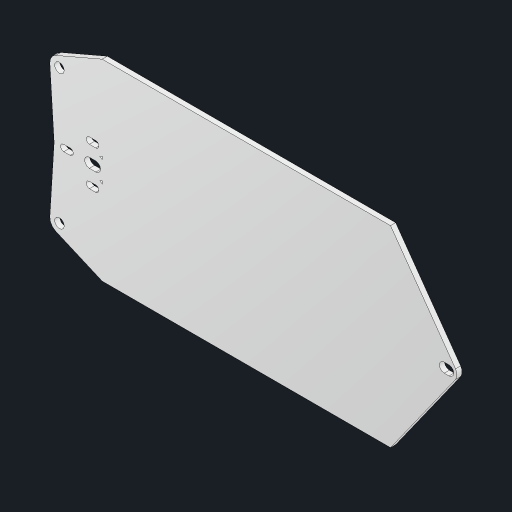
# Autodesk Inventor part: Bottom Plate Poly
Saved by Autodesk Inventor 2023.2 (Build 272271030, 271C)
## iProperties
Created: 2024-02-28
Part Number: Bottom Plate Poly
Material: Aluminum 6061
Document SubType Name: Modeling
Designer: robpl
Density: 2.7 g/cm^3
Appearance: Aluminum - Flat
Mass: 11.953 g
Surface Area: 75.4446 cm^2
Volume: 4.42704 cm^3
Author: robpl
Autodesk Inventor part; units mm, degrees
ref_plane "YZ Plane" through (0, 0, 0) normal (1, 0, 0) x (0, 1, 0)
ref_plane "XZ Plane" through (0, 0, 0) normal (0, 1, 0) x (-1, 0, 0)
ref_plane "XY Plane" through (0, 0, 0) normal (0, 0, 1) x (1, 0, 0)
sketch "Sketch1" plane through (0, 0, 0) normal (0, 0, 1) x (1, 0, 0)
  line L0 (-45, 25) -> (45, 25)
  line L1 (45, 25) -> (45, -25)
  line L2 (45, -25) -> (-45, -25)
  line L3 (-45, -25) -> (-45, 25)
  line L4 (-45, 25) -> (45, -25) construction
  line L5 (45, 25) -> (-45, -25) construction
  line L6 (-45, -25) -> (-40, -25)
  line L7 (-40, -25) -> (-40, -47)
  line L8 (-40, -47) -> (-45, -47)
  line L9 (-45, -47) -> (-45, -25)
  line L10 (45, -25) -> (40, -25)
  line L11 (40, -25) -> (40, -47)
  line L12 (40, -47) -> (45, -47)
  line L13 (45, -47) -> (45, -25)
  line L14 (45, 25) -> (40, 25)
  line L15 (40, 25) -> (40, 47)
  line L16 (40, 47) -> (45, 47)
  line L17 (45, 47) -> (45, 25)
  line L18 (-45, 25) -> (-40, 25)
  line L19 (-40, 25) -> (-40, 47)
  line L20 (-40, 47) -> (-45, 47)
  line L21 (-45, 47) -> (-45, 25)
  circle A0 centre (-48, 0) radius 18
  circle A1 centre (0, 0) radius 66
  circle A2 centre (-58.3352, 21) radius 4
  circle A3 centre (-58.3352, -21) radius 4
  circle A4 centre (-58.3352, -21) radius 1.5
  circle A5 centre (-58.3352, 21) radius 1.5
  line L22 (61.75, 0) -> (63.25, 0) construction
  line L23 (61.75, -4) -> (63.25, -4)
  line L24 (63.25, 4) -> (61.75, 4)
  arc A6 (61.75, 4) -> (61.75, -4) centre (61.75, 0) ccw
  arc A7 (63.25, -4) -> (63.25, 4) centre (63.25, 0) ccw
  line L25 (61.75, 0) -> (63.25, 0) construction
  line L26 (61.75, -1.5) -> (63.25, -1.5)
  line L27 (63.25, 1.5) -> (61.75, 1.5)
  arc A8 (61.75, 1.5) -> (61.75, -1.5) centre (61.75, 0) ccw
  arc A9 (63.25, -1.5) -> (63.25, 1.5) centre (63.25, 0) ccw
  circle A10 centre (61.75, 0) radius 4.25 construction
  circle A11 centre (61.75, 0) radius 4 construction
  line L28 (-45, -25) -> (45, -25) construction
  line L29 (45, -25) -> (45, -30) construction
  line L30 (45, -30) -> (-45, -30)
  line L31 (-45, -30) -> (-45, -25) construction
  line L32 (-45, 30) -> (45, 30)
  line L33 (-47, 0) -> (-49, 0) construction
  line L34 (-47, 1.5) -> (-49, 1.5)
  line L35 (-49, -1.5) -> (-47, -1.5)
  arc A12 (-47, -1.5) -> (-47, 1.5) centre (-47, 0) ccw
  arc A13 (-49, 1.5) -> (-49, -1.5) centre (-49, 0) ccw
  line L36 (-40, 0) -> (-56, 0) construction
  line L37 (-48, -6) -> (-48, 6) construction
  line L38 (-47, 6) -> (-49, 6) construction
  line L39 (-47, 7) -> (-49, 7)
  line L40 (-49, 5) -> (-47, 5)
  arc A14 (-47, 5) -> (-47, 7) centre (-47, 6) ccw
  arc A15 (-49, 7) -> (-49, 5) centre (-49, 6) ccw
  line L41 (-55, 0) -> (-57, 0) construction
  line L42 (-55, 1) -> (-57, 1)
  line L43 (-57, -1) -> (-55, -1)
  arc A16 (-55, -1) -> (-55, 1) centre (-55, 0) ccw
  arc A17 (-57, 1) -> (-57, -1) centre (-57, 0) ccw
  line L44 (-47, -6) -> (-49, -6) construction
  line L45 (-47, -5) -> (-49, -5)
  line L46 (-49, -7) -> (-47, -7)
  arc A18 (-47, -7) -> (-47, -5) centre (-47, -6) ccw
  arc A19 (-49, -5) -> (-49, -7) centre (-49, -6) ccw
  line L47 (-49, 3) -> (-47, 3)
  arc A20 (-47, 3) -> (-47, 9) centre (-47, 6) ccw
  line L48 (-47, 9) -> (-49, 9)
  arc A21 (-49, 9) -> (-49, 3) centre (-49, 6) ccw
  line L49 (-49, -3.5) -> (-47, -3.5)
  arc A22 (-47, -3.5) -> (-47, 3.5) centre (-47, 0) ccw
  line L50 (-47, 3.5) -> (-49, 3.5)
  arc A23 (-49, 3.5) -> (-49, -3.5) centre (-49, 0) ccw
  line L51 (-49, -9) -> (-47, -9)
  arc A24 (-47, -9) -> (-47, -3) centre (-47, -6) ccw
  line L52 (-47, -3) -> (-49, -3)
  arc A25 (-49, -3) -> (-49, -9) centre (-49, -6) ccw
  line L53 (-57, -3) -> (-55, -3)
  arc A26 (-55, -3) -> (-55, 3) centre (-55, 0) ccw
  line L54 (-55, 3) -> (-57, 3)
  arc A27 (-57, 3) -> (-57, -3) centre (-57, 0) ccw
  line L55 (-40, 25) -> (-44.0624, 5.3914)
  line L56 (-40, -25) -> (-44.0624, -5.3914)
  line L57 (61.75, -2.5) -> (63.25, -2.5)
  arc A28 (63.25, -2.5) -> (63.25, 2.5) centre (63.25, 0) ccw
  line L58 (63.25, 2.5) -> (61.75, 2.5)
  arc A29 (61.75, 2.5) -> (61.75, -2.5) centre (61.75, 0) ccw
  line L59 (65.2879, -1.4481) -> (45, -30)
  line L60 (45, 30) -> (65.2879, 1.4481)
  line L61 (42.4191, 25) -> (59.464, 1.0121)
  line L62 (42.4191, -25) -> (59.464, -1.0121)
  circle A30 centre (-58.3352, -21) radius 3
  circle A31 centre (-58.3352, 21) radius 3
  line L63 (-45, -30) -> (-59.5204, -23.756)
  line L64 (-45, 30) -> (-59.5204, 23.756)
  line L65 (-60, 0) -> (-61.3291, -20.8088)
  line L66 (-60, 0) -> (-61.3291, 20.8088)
  point P0 (62.5, 0)
  point P1 (62.5, 0)
  point P2 (-45.7543, -3.2708)
  point P3 (-45.7543, 3.2708)
  point P4 (58.5132, -2.3502)
  point P5 (58.5132, 2.3502)
  point P6 (-45, 3.7639)
  point P7 (-45, 2.8723)
  point P8 (-45, -2.8723)
  point P9 (-45, -3.7639)
  dimension "d0" = 90
  dimension "d1" = 50
  dimension "d2" = 5
  dimension "d3" = 22
  dimension "d5" = 36
  dimension "d6" = 132
  dimension "d7" = 8
  dimension "d8" = 8
  dimension "d9" = 4
  dimension "d10" = 3
  dimension "d11" = 3
  dimension "d12" = 8
  dimension "d13" = 3
  dimension "d14" = 1.5
  dimension "d15" = 8.5
  dimension "d16" = 1.25
  dimension "d17" = 5
  dimension "d18" = 5
  dimension "d19" = 1
  dimension "d20" = 3
  dimension "d21" = 16
  dimension "d22" = 12
  dimension "d23" = 1
  dimension "d24" = 1
  dimension "d25" = 1
  dimension "d26" = 2
  dimension "d27" = 1
  dimension "d28" = 2
  dimension "d29" = 2
  dimension "d30" = 2
  dimension "d31" = 2
  dimension "d32" = 2
  dimension "d33" = 1
  dimension "d35" = 5
  dimension "d36" = 5
  dimension "d37" = 1.5
  dimension "d38" = 1.5
  constraints: 146 end point, 55 point on circle, 36 tangent, 31 centre point, 26 parallel, 11 horizontal, 10 midpoint, 8 perpendicular, 6 coincident, 6 point on line, 5 equal length, 2 horizontal alignment, 2 vertical alignment, 1 collinear, 17 other
  measures "d0" distance of L1.end L2.end
  measures "d1" distance of L0.end L1.end
  measures "d2" distance of L7.end L8.end
  measures "d3" distance of L6.end L7.end
  measures "d5" diameter of A0
  measures "d6" diameter of A1
  measures "d7" diameter of A2
  measures "d8" diameter of A3
  measures "d9" distance from line of A2.centre L0
  measures "d10" diameter of A4
  measures "d11" diameter of A5
  measures "d12" diameter of A7
  measures "d13" diameter of A9
  measures "d14" distance of L22.start L22.end
  measures "d15" diameter of A10
  measures "d17" distance of L28.end L29.end
  measures "d18" distance from line of L14.end L32
  measures "d19" distance of A0.centre L33.end
  measures "d20" diameter of A13
  measures "d21" distance of L36.start L36.end
  measures "d22" distance of L37.start L37.end
  measures "d23" distance of L37.end L38.end
  measures "d24" radius of A15
  measures "d25" distance of L36.end L41.end
  measures "d26" diameter of A17
  measures "d27" distance of L37.start L44.end
  measures "d28" diameter of A19
  measures "d29" radial gap between concentric circles of A15 A21
  measures "d30" radial gap between concentric circles of A13 A23
  measures "d31" radial gap between concentric circles of A19 A25
  measures "d32" radial gap between concentric circles of A17 A27
  measures "d33" radial gap between concentric circles of A8 A29
  measures "d35" distance between parallel lines of L60 L61
  measures "d36" distance between parallel lines of L59 L62
  measures "d37" radial gap between concentric circles of A4 A30
  measures "d38" radial gap between concentric circles of A5 A31
extrude "Extrusion1" add sketch "Sketch1" along normal blind 1.6 contours L21 L32 L19 L0 | L0 L55 A0 L3 | L3 A0 L66 A2 L64 L21 | L19 L32 L15 L0 | L0 L61 L1 L62 L2 L56 A0 L55 | A0 L55 A20 L3 | L3 A20 L48 A21 A23 A26 L54 A27 L66 A0 | L15 L32 L17 L0 | A0 L56 A24 L3 A22 A20 L55 | A20 L3 | L3 A20 A22 L50 A23 A21 L48 | A2 L66 A31 L64 | L0 L1 L61 | A27 L54 A26 A23 L53 | A27 L53 A26 A23 A25 L51 A24 L3 A0 L65 | A31 | L17 L60 A7 L24 A6 L61 L1 | L61 A6 L62 L1 | L56 L2 L3 A0 | A0 L3 A24 L56 | A22 L3 | L3 A22 A24 L52 A25 A23 A26 A21 L47 A20 | A20 L47 A21 A23 L50 A22 | A0 L3 L9 L63 A3 L65 | L62 A6 L23 A7 L59 L13 L1 | L1 L2 L62 | L61 A29 L62 A6 | A6 L24 A7 L60 A28 L58 A29 L61 | L7 L30 L9 L2 | L2 L11 L30 L7 | A24 L3 | A3 L63 A30 L65 | L13 L30 L11 L2 | L62 A29 L57 A28 L59 A7 L23 A6 | A29 L58 A28 L57 | A24 L51 A25 A23 L49 A22 L3 | A22 L49 A23 A25 L52 A24 | A26 A23 | A30 picked at (-54.7053, 20.6889) picked at (-54.7053, -20.6889)
sketch "Sketch2" plane through (0, 0, 0) normal (0, 0, -1) x (-1, 0, 0)
  line L0 (-45, -30) -> (-65.2879, -1.4481) projected
  line L1 (45, -30) -> (-45, -30) projected
  line L2 (59.5204, -23.756) -> (45, -30) projected
  arc A0 (59.5204, -23.756) -> (61.3291, -20.8088) centre (58.3352, -21) ccw projected
  line L3 (60, 0) -> (61.3291, -20.8088) projected
  line L4 (61.3291, 20.8088) -> (60, 0) projected
  arc A1 (61.3291, 20.8088) -> (59.5204, 23.756) centre (58.3352, 21) ccw projected
  line L5 (45, 30) -> (59.5204, 23.756) projected
  line L6 (-45, 30) -> (45, 30) projected
  line L7 (-65.2879, 1.4481) -> (-45, 30) projected
  arc A2 (-65.2879, 1.4481) -> (-65.2879, -1.4481) centre (-63.25, 0) ccw projected
  arc A3 (45, 3.7639) -> (45.7543, 3.2708) centre (47, 6) ccw projected
  arc A4 (45, -2.8723) -> (45.7543, -3.2708) centre (47, 0) ccw projected
  arc A5 (45.7543, -3.2708) -> (45, -3.7639) centre (47, -6) ccw projected
  arc A6 (55, 1) -> (55, -1) centre (55, 0) ccw projected
  line L8 (57, 1) -> (55, 1) projected
  arc A7 (57, -1) -> (57, 1) centre (57, 0) ccw projected
  line L9 (55, -1) -> (57, -1) projected
  arc A8 (47, 7) -> (47, 5) centre (47, 6) ccw projected
  line L10 (49, 7) -> (47, 7) projected
  arc A9 (49, 5) -> (49, 7) centre (49, 6) ccw projected
  line L11 (47, 5) -> (49, 5) projected
  arc A10 (47, 1.5) -> (47, -1.5) centre (47, 0) ccw projected
  line L12 (49, 1.5) -> (47, 1.5) projected
  arc A11 (49, -1.5) -> (49, 1.5) centre (49, 0) ccw projected
  line L13 (47, -1.5) -> (49, -1.5) projected
  arc A12 (47, -5) -> (47, -7) centre (47, -6) ccw projected
  line L14 (49, -5) -> (47, -5) projected
  arc A13 (49, -7) -> (49, -5) centre (49, -6) ccw projected
  line L15 (47, -7) -> (49, -7) projected
  circle A14 centre (58.3352, 21) radius 1.5 projected
  circle A15 centre (58.3352, -21) radius 1.5 projected
  arc A16 (-61.75, -1.5) -> (-61.75, 1.5) centre (-61.75, 0) ccw projected
  line L16 (-63.25, -1.5) -> (-61.75, -1.5) projected
  arc A17 (-63.25, 1.5) -> (-63.25, -1.5) centre (-63.25, 0) ccw projected
  line L17 (-61.75, 1.5) -> (-63.25, 1.5) projected
  line L18 (-44.2249, 32.3768) -> (-45.7751, 27.6232)
  line L19 (-45.7751, 27.6232) -> (46.2249, -2.3768)
  line L20 (46.2249, -2.3768) -> (47.7751, 2.3768)
  line L21 (47.7751, 2.3768) -> (-44.2249, 32.3768)
  line L22 (-45.7751, -27.6232) -> (-44.2249, -32.3768)
  line L23 (-44.2249, -32.3768) -> (47.7751, -2.3768)
  line L24 (47.7751, -2.3768) -> (46.2249, 2.3768)
  line L25 (46.2249, 2.3768) -> (-45.7751, -27.6232)
  line L26 (40, 25) -> (-42.4191, 25) projected
  line L27 (-44.9191, 25) -> (-39.9191, 25)
  line L28 (-39.9191, 25) -> (-39.9191, -25)
  line L29 (-39.9191, -25) -> (-44.9191, -25)
  line L30 (-44.9191, -25) -> (-44.9191, 25)
  line L31 (45, -2.8723) -> (45, -3.7639) projected
  arc A18 (45.7543, 3.2708) -> (45, 2.8723) centre (47, 0) ccw projected
  line L32 (45, 3.7639) -> (45, 2.8723) projected
  point P0 (0, 0)
  point P1 (-42.4191, -25)
  point P2 (38.936, 0)
  point P3 (-21.6027, 25)
  point P4 (45.4462, 3.1362)
  point P5 (45.4462, -3.1362)
  point P6 (-37.7306, 25)
  point P7 (43.8961, 1.6174)
  point P8 (43.8961, -1.6174)
  point P9 (-36.936, -30)
  point P10 (-36.936, 30)
  point P11 (45, -3.2817)
  dimension "d42" = 5
  constraints: 24 end point, 6 midpoint, 6 parallel, 3 perpendicular, 2 equal length, 1 coincident, 1 point on line
  measures "d42" distance of L19.end L20.end
extrude "Extrusion2" [suppressed]
sketch "Sketch3" plane through (0, 0, 0) normal (0, 0, -1) x (-1, 0, 0)
  arc A0 (45, -2.8723) -> (45.7543, -3.2708) centre (47, 0) ccw projected
  arc A1 (45.7543, -3.2708) -> (45, -3.7639) centre (47, -6) ccw projected
  arc A2 (45, 3.7639) -> (45.7543, 3.2708) centre (47, 6) ccw projected
  arc A3 (-61.75, -1.5) -> (-61.75, 1.5) centre (-61.75, 0) ccw projected
  line L0 (-63.25, -1.5) -> (-61.75, -1.5) projected
  arc A4 (-63.25, 1.5) -> (-63.25, -1.5) centre (-63.25, 0) ccw projected
  line L1 (-61.75, 1.5) -> (-63.25, 1.5) projected
  circle A5 centre (58.3352, -21) radius 1.5 projected
  circle A6 centre (58.3352, 21) radius 1.5 projected
  arc A7 (47, -5) -> (47, -7) centre (47, -6) ccw projected
  line L2 (49, -5) -> (47, -5) projected
  arc A8 (49, -7) -> (49, -5) centre (49, -6) ccw projected
  line L3 (47, -7) -> (49, -7) projected
  arc A9 (47, 1.5) -> (47, -1.5) centre (47, 0) ccw projected
  line L4 (49, 1.5) -> (47, 1.5) projected
  arc A10 (49, -1.5) -> (49, 1.5) centre (49, 0) ccw projected
  line L5 (47, -1.5) -> (49, -1.5) projected
  arc A11 (47, 7) -> (47, 5) centre (47, 6) ccw projected
  line L6 (49, 7) -> (47, 7) projected
  arc A12 (49, 5) -> (49, 7) centre (49, 6) ccw projected
  line L7 (47, 5) -> (49, 5) projected
  arc A13 (55, 1) -> (55, -1) centre (55, 0) ccw projected
  line L8 (57, 1) -> (55, 1) projected
  arc A14 (57, -1) -> (57, 1) centre (57, 0) ccw projected
  line L9 (55, -1) -> (57, -1) projected
  line L10 (-45, 30) -> (45, 30) projected
  line L11 (-65.2879, 1.4481) -> (-45, 30) projected
  arc A15 (-65.2879, 1.4481) -> (-65.2879, -1.4481) centre (-63.25, 0) ccw projected
  line L12 (-45, -30) -> (-65.2879, -1.4481) projected
  line L13 (45, -30) -> (-45, -30) projected
  line L14 (59.5204, -23.756) -> (45, -30) projected
  arc A16 (59.5204, -23.756) -> (61.3291, -20.8088) centre (58.3352, -21) ccw projected
  line L15 (60, 0) -> (61.3291, -20.8088) projected
  line L16 (61.3291, 20.8088) -> (60, 0) projected
  arc A17 (61.3291, 20.8088) -> (59.5204, 23.756) centre (58.3352, 21) ccw projected
  line L17 (45, 30) -> (59.5204, 23.756) projected
  circle A18 centre (58.3352, -21) radius 4.5
  arc A19 (49, -10) -> (49, -2) centre (49, -6) ccw
  line L18 (49, -2) -> (47, -2)
  arc A20 (47, -2) -> (47, -10) centre (47, -6) ccw
  line L19 (47, -10) -> (49, -10)
  arc A21 (57, -4) -> (57, 4) centre (57, 0) ccw
  line L20 (57, 4) -> (55, 4)
  arc A22 (55, 4) -> (55, -4) centre (55, 0) ccw
  line L21 (55, -4) -> (57, -4)
  line L22 (58.3352, -21) -> (44.3823, -27)
  line L23 (44.3823, -27) -> (-43.4515, -27)
  line L24 (-43.4515, -27) -> (-62.6366, 0)
  line L25 (-62.6366, 0) -> (-43.4515, 27)
  line L26 (-43.4515, 27) -> (44.3823, 27)
  line L27 (44.3823, 27) -> (58.3352, 21)
  line L28 (58.3352, 21) -> (56.9939, 0)
  line L29 (56.9939, 0) -> (58.3352, -21)
  line L30 (48.4499, 0.9987) -> (-40.4795, -28)
  line L31 (-40.4795, -28) -> (42.4422, -28)
  line L32 (42.4422, -28) -> (48.4499, 0.9987)
  circle A23 centre (55.191, -6.194) radius 2.194
  line L33 (45, -2.8723) -> (45, -3.7639) projected
  arc A24 (45.7543, 3.2708) -> (45, 2.8723) centre (47, 0) ccw projected
  line L34 (45, 3.7639) -> (45, 2.8723) projected
  point P0 (0, 0)
  point P1 (46.1885, -9.9168)
  point P2 (42.6494, -27)
  point P3 (54.2013, -22.7777)
  point P4 (58.0484, -16.5092)
  point P5 (57.3806, -6.0542)
  point P6 (52.998, -6.1253)
  dimension "d45" = 3
  dimension "d46" = 3
  dimension "d47" = 3
  dimension "d48" = 3
  constraints: 30 end point, 8 point on circle, 6 centre point, 3 tangent, 13 other
  measures "d45" radial gap between concentric circles of A5 A18
  measures "d46" distance between parallel lines of L3 L19
  measures "d47" distance between parallel lines of L9 L21
  measures "d48" distance between parallel lines of L15 L29
extrude "Extrusion3" [suppressed]
mirror "Mirror1" [suppressed]
fillet "Fillet2" [suppressed]
sketch "Sketch4" plane through (0, 0, 1.6) normal (0, 0, 1) x (1, 0, 0)
  line L0 (-22.0827, 1.5) -> (-35.6504, 1.5)
  line L1 (-35.6504, 1.5) -> (-42.4343, 13.25)
  line L2 (-42.4343, 13.25) -> (-35.6504, 25)
  line L3 (-35.6504, 25) -> (-22.0827, 25)
  line L4 (-22.0827, 25) -> (-15.2988, 13.25)
  line L5 (-15.2988, 13.25) -> (-22.0827, 1.5)
  line L6 (7.6508, 0) -> (0.867, -11.75)
  line L7 (0.867, -11.75) -> (-12.7007, -11.75)
  line L8 (-12.7007, -11.75) -> (-19.4846, 0)
  line L9 (-19.4846, 0) -> (-12.7007, 11.75)
  line L10 (-12.7007, 11.75) -> (0.867, 11.75)
  line L11 (0.867, 11.75) -> (7.6508, 0)
  line L12 (-15.2988, -13.25) -> (-22.0827, -25)
  line L13 (-22.0827, -25) -> (-35.6504, -25)
  line L14 (-35.6504, -25) -> (-42.4343, -13.25)
  line L15 (-42.4343, -13.25) -> (-35.6504, -1.5)
  line L16 (-35.6504, -1.5) -> (-22.0827, -1.5)
  line L17 (-22.0827, -1.5) -> (-15.2988, -13.25)
  line L18 (-38.3719, 25) -> (42.4191, 25) projected
  line L19 (42.4191, -25) -> (-38.3719, -25) projected
  line L20 (-44.0624, 5.3914) -> (-40.3303, 23.4057) projected
  line L21 (-40.3303, -23.4057) -> (-44.0624, -5.3914) projected
  line L22 (7.6508, 26.5) -> (0.867, 14.75)
  line L23 (0.867, 14.75) -> (-12.7007, 14.75)
  line L24 (-12.7007, 14.75) -> (-19.4846, 26.5)
  line L25 (-19.4846, 26.5) -> (-12.7007, 38.25)
  line L26 (-12.7007, 38.25) -> (0.867, 38.25)
  line L27 (0.867, 38.25) -> (7.6508, 26.5)
  line L28 (0.867, -38.25) -> (-12.7007, -38.25)
  line L29 (-12.7007, -38.25) -> (-19.4846, -26.5)
  line L30 (-19.4846, -26.5) -> (-12.7007, -14.75)
  line L31 (-12.7007, -14.75) -> (0.867, -14.75)
  line L32 (0.867, -14.75) -> (7.6508, -26.5)
  line L33 (7.6508, -26.5) -> (0.867, -38.25)
  line L34 (24.2428, 1.5) -> (10.2489, 1.5)
  line L35 (10.2489, 1.5) -> (3.252, 13.6191)
  line L36 (3.252, 13.6191) -> (10.2489, 25.7381)
  line L37 (10.2489, 25.7381) -> (24.2428, 25.7381)
  line L38 (24.2428, 25.7381) -> (31.2398, 13.6191)
  line L39 (31.2398, 13.6191) -> (24.2428, 1.5)
  line L40 (26.4154, 0) -> (33.1993, 11.75)
  line L41 (30.6012, 13.25) -> (23.8173, 1.5)
  line L42 (23.8173, 1.5) -> (10.2496, 1.5)
  line L43 (23.8173, 25) -> (30.6012, 13.25)
  line L44 (10.2496, 25) -> (23.8173, 25)
  line L45 (33.1993, -11.75) -> (26.4154, 0)
  line L46 (23.8173, -1.5) -> (30.6012, -13.25)
  line L47 (33.1993, 11.75) -> (46.767, 11.75)
  line L48 (46.767, 11.75) -> (53.5508, 0)
  line L49 (46.767, -11.75) -> (33.1993, -11.75)
  line L50 (33.1993, -14.75) -> (46.767, -14.75)
  line L51 (30.6012, -13.25) -> (23.8173, -25)
  line L52 (26.4154, -26.5) -> (33.1993, -14.75)
  line L53 (53.5508, 0) -> (46.767, -11.75)
  line L54 (46.767, -14.75) -> (53.5508, -26.5)
  line L55 (10.2496, 1.5) -> (3.4657, 13.25)
  line L56 (3.4657, 13.25) -> (10.2496, 25)
  line L57 (10.2496, -1.5) -> (23.8173, -1.5)
  line L58 (23.8173, -25) -> (10.2496, -25)
  line L59 (3.4657, -13.25) -> (10.2496, -1.5)
  line L60 (10.2496, -25) -> (3.4657, -13.25)
  line L61 (53.5508, -26.5) -> (46.767, -38.25)
  line L62 (46.767, -38.25) -> (33.1993, -38.25)
  line L63 (33.1993, -38.25) -> (26.4154, -26.5)
  line L64 (33.1993, 14.75) -> (26.4154, 26.5)
  line L65 (53.5508, 26.5) -> (46.767, 14.75)
  line L66 (46.767, 38.25) -> (53.5508, 26.5)
  line L67 (33.1993, 38.25) -> (46.767, 38.25)
  line L68 (26.4154, 26.5) -> (33.1993, 38.25)
  line L69 (46.767, 14.75) -> (33.1993, 14.75)
  line L70 (45, -30) -> (65.2879, -1.4481) projected
  arc A0 (65.2879, -1.4481) -> (65.2879, 1.4481) centre (63.25, 0) ccw projected
  line L71 (65.2879, 1.4481) -> (45, 30) projected
  line L72 (45, 30) -> (-45, 30) projected
  line L73 (-45, 30) -> (-59.5204, 23.756) projected
  arc A1 (-59.5204, 23.756) -> (-61.3291, 20.8088) centre (-58.3352, 21) ccw projected
  line L74 (-61.3291, 20.8088) -> (-60, 0) projected
  line L75 (-60, 0) -> (-61.3291, -20.8088) projected
  arc A2 (-61.3291, -20.8088) -> (-59.5204, -23.756) centre (-58.3352, -21) ccw projected
  line L76 (-59.5204, -23.756) -> (-45, -30) projected
  line L77 (-45, -30) -> (45, -30) projected
  arc A3 (-55, -1) -> (-55, 1) centre (-55, 0) ccw projected
  line L78 (-55, -1) -> (-57, -1) projected
  arc A4 (-57, 1) -> (-57, -1) centre (-57, 0) ccw projected
  line L79 (-57, 1) -> (-55, 1) projected
  arc A5 (-47, 5) -> (-47, 7) centre (-47, 6) ccw projected
  line L80 (-47, 5) -> (-49, 5) projected
  arc A6 (-49, 7) -> (-49, 5) centre (-49, 6) ccw projected
  line L81 (-49, 7) -> (-47, 7) projected
  arc A7 (-47, -1.5) -> (-47, 1.5) centre (-47, 0) ccw projected
  line L82 (-47, -1.5) -> (-49, -1.5) projected
  arc A8 (-49, 1.5) -> (-49, -1.5) centre (-49, 0) ccw projected
  line L83 (-49, 1.5) -> (-47, 1.5) projected
  arc A9 (-47, -7) -> (-47, -5) centre (-47, -6) ccw projected
  line L84 (-47, -7) -> (-49, -7) projected
  arc A10 (-49, -5) -> (-49, -7) centre (-49, -6) ccw projected
  line L85 (-49, -5) -> (-47, -5) projected
  circle A11 centre (-58.3352, 21) radius 1.5 projected
  circle A12 centre (-58.3352, -21) radius 1.5 projected
  arc A13 (61.75, 1.5) -> (61.75, -1.5) centre (61.75, 0) ccw projected
  line L86 (61.75, 1.5) -> (63.25, 1.5) projected
  arc A14 (63.25, -1.5) -> (63.25, 1.5) centre (63.25, 0) ccw projected
  line L87 (63.25, -1.5) -> (61.75, -1.5) projected
  line L88 (-45, -2.8723) -> (-45, -3.7639) projected
  line L89 (-45, 3.7639) -> (-45, 2.8723) projected
  arc A15 (-45, -3.7639) -> (-45.7543, -3.2708) centre (-47, -6) ccw projected
  arc A16 (-45.7543, -3.2708) -> (-45, -2.8723) centre (-47, 0) ccw projected
  arc A17 (-45, 2.8723) -> (-45.7543, 3.2708) centre (-47, 0) ccw projected
  arc A18 (-45.7543, 3.2708) -> (-45, 3.7639) centre (-47, 6) ccw projected
  point P0 (0, 0)
  point P1 (-28.8666, 13.25)
  point P2 (-5.9169, 0)
  point P3 (-28.8666, -13.25)
  point P4 (-5.9169, 26.5)
  point P5 (-5.9169, -26.5)
  point P6 (17.2459, 13.6191)
  point P7 (6.7504, 7.5595)
  point P8 (17.0334, 13.25)
  point P9 (39.9831, 0)
  point P10 (17.0334, -13.25)
  point P11 (39.9831, -26.5)
  point P12 (39.9831, 26.5)
  point P13 (52.6504, 7.5595)
  point P14 (49.152, 13.6191)
  point P15 (-18.6186, -25)
  point P16 (6.7848, -25)
  point P17 (27.2814, -25)
  point P18 (27.2814, 25)
  point P19 (24.669, 25)
  point P20 (9.8228, 25)
  point P21 (6.7848, 25)
  point P22 (-18.6186, 25)
  dimension "d54" = 3
  dimension "d55" = 3
  dimension "d56" = 3
  dimension "d57" = 3
  dimension "d58" = 3
  dimension "d59" = 3
  dimension "d60" = 3
  dimension "d61" = 32.3316
  dimension "d64" = 45.9
  constraints: 132 end point, 6 horizontal, 4 equal length, 3 collinear, 2 point on line, 1 horizontal alignment, 1 midpoint, 145 other
  measures "d54" distance between parallel lines of L0 L16
  measures "d55" distance between parallel lines of L5 L9
  measures "d56" distance between parallel lines of L4 L24
  measures "d57" distance between parallel lines of L10 L23
  measures "d58" distance between parallel lines of L12 L30
  measures "d59" distance between parallel lines of L7 L31
  measures "d60" distance from line of L11 point (6.75, 7.56)
  measures "d61" distance of L0.start L34.end
  measures "d64" distance of L8.end L40.start
extrude "Extrusion4" [suppressed]
equation "\"d15\" = d12 + 0.333333 * d14"
equation "\"d18\" = d17"
equation "\"d35\" = d34"
equation "\"d34\" = d17"
body "Solid1"
